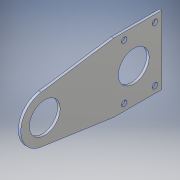
# Autodesk Inventor part: CAR_041_KickerGusset
Saved by Autodesk Inventor 2018.3 (Build 223284000, 284)
## iProperties
Created: 2020-02-13
Part Number: CAR_041_KickerGusset
Material: Aluminum 6061
Document SubType Name: Modeling
Designer: user
Mass: 30.5753 g
Surface Area: 109.486 cm^2
Volume: 11.3242 cm^3
Density: 2.7 g/cm^3
Appearance: Aluminum - Flat
Author: user
Autodesk Inventor part; units mm, degrees
ref_plane "YZ Plane" through (0, 0, 0) normal (1, 0, 0) x (0, 1, 0)
ref_plane "XZ Plane" through (0, 0, 0) normal (0, 1, 0) x (-1, 0, 0)
ref_plane "XY Plane" through (0, 0, 0) normal (0, 0, 1) x (1, 0, 0)
sketch "Sketch1" plane through (0, 0, 0) normal (1, 0, 0) x (0, 1, 0)
  line L0 (0, 0) -> (63.5, 0)
  line L1 (63.5, 0) -> (63.5, 44.45)
  line L2 (0, 44.45) -> (0, 0)
  line L3 (31.75, 139.6202) -> (31.75, -24.2766) construction
  arc A0 (53.7441, 111.6025) -> (9.7559, 111.6025) centre (31.75, 108.4072) ccw
  line L4 (63.5, 44.45) -> (53.7441, 111.6025)
  line L5 (0, 44.45) -> (9.7559, 111.6025)
  line L6 (0, 22.225) -> (-15.9644, 22.225)
  point P0 (31.75, 25.908)
  dimension "d0" = 63.5
  dimension "d1" = 44.45
  dimension "d3" = 31.75
  dimension "d5" = 44.45
  dimension "d21" = 82.4992
  dimension "d22" = 63.9572
  dimension "d40" = 25.908
  constraints: 14 end point, 2 coincident, 2 horizontal, 2 parallel, 2 point on circle, 2 tangent, 1 centre point, 1 midpoint, 1 perpendicular, 1 point on line, 1 vertical, 1 vertical alignment
  measures "d0" distance of L2.start L1.end
  measures "d1" distance of L2.start L0.start
  measures "d3" distance between parallel lines of L1 L3
  measures "d5" diameter of A0
  measures "d21" distance of point (31.75, 25.908) point (31.75, 108.407)
  measures "d22" vertical distance of L1.end point (31.75, 108.407)
  measures "d40" distance from line of L0 point (31.75, 25.908)
extrude "Extrusion1" add sketch "Sketch1" along normal blind 2.286
hole "Hole2" at (0, 31.75, 108.4072) at (0, 31.75, 25.908) direction (1, 0, 0) diameter 28.575 end through all
sketch "Sketch2" plane through (2.286, 0, 0) normal (1, 0, 0) x (0, 0, -1)
  line L0 (0, 63.5) -> (-44.45, 63.5) projected
  line L1 (-12.7, -16.6387) -> (-12.7, 68.9005) construction
  line L2 (0, 0) -> (0, 63.5) construction
  circle A0 centre (-25.908, 31.75) radius 14.2875 projected
  circle A1 centre (-25.908, 31.75) radius 22.0437
  circle A2 centre (-6.35, 57.15) radius 4.5847
  line L3 (-0.8507, 57.15) -> (-3.6004, 52.3875)
  line L4 (-3.6004, 52.3875) -> (-9.0996, 52.3875)
  line L5 (-9.0996, 52.3875) -> (-11.8493, 57.15)
  line L6 (-11.8493, 57.15) -> (-9.0996, 61.9125)
  line L7 (-9.0996, 61.9125) -> (-3.6004, 61.9125)
  line L8 (-3.6004, 61.9125) -> (-0.8507, 57.15)
  circle A3 centre (-34.925, 57.15) radius 4.5847
  line L9 (-29.631, 57.15) -> (-32.278, 52.5653)
  line L10 (-32.278, 52.5653) -> (-37.572, 52.5653)
  line L11 (-37.572, 52.5653) -> (-40.219, 57.15)
  line L12 (-40.219, 57.15) -> (-37.572, 61.7347)
  line L13 (-37.572, 61.7347) -> (-32.278, 61.7347)
  line L14 (-32.278, 61.7347) -> (-29.631, 57.15)
  point P0 (-6.35, 6.35)
  point P1 (-34.925, 6.35)
  dimension "d33" = 9.1694
  dimension "d35" = 9.525
  dimension "d37" = 25.4
  dimension "d39" = 25.4
  dimension "d41" = 9.525
  dimension "d42" = 38.1
  constraints: 26 end point, 5 coincident, 3 centre point, 3 horizontal alignment, 2 vertical alignment, 1 equal radius, 1 tangent, 1 vertical, 26 other
  measures "d33" diameter of A2
  measures "d35" distance between parallel lines of L4 L7
  measures "d37" vertical distance of A2.centre A0.centre
  measures "d39" vertical distance of point (-6.35, 6.35) A0.centre
  measures "d41" horizontal distance of L0.end point (-34.925, 57.15)
  measures "d42" horizontal distance of A2.centre L0.end
hole "Hole1" at (2.286, 57.15, 34.925) at (2.286, 57.15, 6.35) at (2.286, 6.35, 34.925) at (2.286, 6.35, 6.35) direction (-1, 0, 0) diameter 5.1054 end through all clearance for "Flat Head Machine Screw (82)" size "#10" standard "Ansi Unified Screw Threads"
equation "\"d3\" = 0.5 * d0"
equation "\"d39\" = d37"
body "Solid1"
